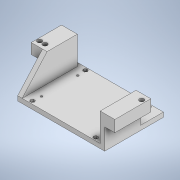
# Autodesk Inventor part: tttray
Saved by Autodesk Inventor 2020 (Build 240168000, 168)
## iProperties
Created: 2022-10-28
Part Number: tttray
Material: 일반
Document SubType Name: Modeling
Designer: SeungJin
Density: 1 g/cm^3
Appearance: 기본값
Author: SeungJin
Autodesk Inventor part; units mm, degrees
ref_plane "YZ Plane" through (0, 0, 0) normal (1, 0, 0) x (0, 1, 0)
ref_plane "XZ Plane" through (0, 0, 0) normal (0, 1, 0) x (-1, 0, 0)
ref_plane "XY Plane" through (0, 0, 0) normal (0, 0, 1) x (1, 0, 0)
sketch "스케치1" plane through (0, 0, 0) normal (0, 1, 0) x (-1, 0, 0)
  line L0 (96.25, 0) -> (-96.25, 0)
  line L1 (-96.25, 0) -> (-96.25, 67)
  line L2 (-96.25, 67) -> (96.25, 67)
  line L3 (96.25, 67) -> (96.25, 0)
  line L4 (96.25, 0) -> (-96.25, 0)
  line L5 (-96.25, 0) -> (-96.25, -63)
  line L6 (-96.25, -63) -> (96.25, -63)
  line L7 (96.25, -63) -> (96.25, 0)
  point P0 (0, 0)
  point P1 (0, 0)
  dimension "d0" = 192.5
  dimension "d1" = 67
  dimension "d2" = 192.5
  dimension "d3" = 63
  constraints: 16 end point, 4 parallel, 2 coincident, 2 horizontal, 2 perpendicular, 1 midpoint
  measures "d0" distance of L1.end L2.end
  measures "d1" distance of L2.end L0.start
  measures "d2" distance of L6.end L5.end
  measures "d3" distance of L6.end L0.start
extrude "돌출1" add sketch "스케치1" along normal blind 10
sketch "스케치2" plane through (0, 10, 0) normal (0, 1, 0) x (1, 0, 0)
  line L0 (-96.25, 0) -> (96.25, 0) projected
  line L1 (-96.25, -67) -> (96.25, -67) projected
  line L2 (86.25, -67) -> (86.25, 12.5)
  line L3 (96.25, -67) -> (96.25, 63) projected
  line L4 (96.25, 12.5) -> (86.25, 12.5)
  line L5 (-86.25, -67) -> (-86.25, 55)
  line L6 (-96.25, 63) -> (-96.25, -67) projected
  line L7 (-96.25, 55) -> (-86.25, 55)
  point P0 (0, 0)
  dimension "d6" = 10
  dimension "d7" = 12.5
  dimension "d8" = 10
  dimension "d9" = 55
  constraints: 8 end point, 4 point on line, 2 perpendicular, 2 vertical
  measures "d6" distance between parallel lines of L2 L3
  measures "d7" distance between parallel lines of L4 L0
  measures "d8" distance between parallel lines of L6 L5
  measures "d9" distance between parallel lines of L7 L0
extrude "돌출2" add sketch "스케치2" along normal blind 62 contours L6 L7 L5 L0 | L0 L5 L1 L6 | L2 L4 L3 L0 | L0 L3 L1 L2
sketch "스케치3" plane through (0, 72, 0) normal (0, 1, 0) x (1, 0, 0)
  line L0 (96.25, -67) -> (96.25, 12.5) projected
  line L1 (96.25, 12.5) -> (86.25, 12.5) projected
  line L2 (86.25, 12.5) -> (86.25, -67) projected
  line L3 (86.25, -67) -> (96.25, -67) projected
  line L4 (96.25, -67) -> (118.75, -67)
  line L5 (118.75, -67) -> (118.75, 12.5)
  line L6 (118.75, 12.5) -> (96.25, 12.5)
  line L7 (96.25, 12.5) -> (96.25, -67)
  point P0 (0, 0)
  dimension "d12" = 22.5
  constraints: 8 end point, 2 parallel, 1 horizontal, 1 perpendicular
  measures "d12" distance of L6.end L5.end
extrude "돌출3" add sketch "스케치3" against normal blind 25.3 contours L0 L6 L5 L4
sketch "스케치5" plane through (0, 72, 0) normal (0, 1, 0) x (1, 0, 0)
  line L0 (-96.25, 55) -> (-96.25, -67) projected
  line L1 (-96.25, -67) -> (-86.25, -67) projected
  line L2 (-86.25, -67) -> (-86.25, 55) projected
  line L3 (-86.25, 55) -> (-96.25, 55) projected
  line L4 (-96.25, 63) -> (-96.25, 55) projected
  line L5 (-96.25, 55) -> (-121.25, 55)
  line L6 (-121.25, 55) -> (-121.25, -12)
  line L7 (-121.25, -12) -> (-96.25, -12)
  line L8 (-96.25, -12) -> (-96.25, 55)
  line L9 (-96.25, 0) -> (96.25, 0) projected
  point P0 (0, 0)
  dimension "d15" = 25
  dimension "d16" = 12
  constraints: 8 end point, 2 parallel, 1 horizontal, 1 perpendicular
  measures "d15" distance between parallel lines of L6 L0
  measures "d16" distance between parallel lines of L9 L7
extrude "돌출4" add sketch "스케치5" against normal blind 23 contours L0 L7 L6 L5
sketch "스케치6" plane through (0, 72, 0) normal (0, 1, 0) x (1, 0, 0)
  line L0 (-96.25, 0) -> (96.25, 0) projected
  line L1 (86.25, 12.5) -> (86.25, -67) projected
  point P0 (0, 0)
  point P1 (111.25, 0)
  point P2 (-114.75, 0)
  point P3 (-102.75, 0)
  dimension "d19" = 25
  dimension "d20" = 214
  dimension "d21" = 12
  measures "d19" distance from line of point (111.25, 0) L1
  measures "d20" distance of point (-102.75, 0) point (111.25, 0)
  measures "d21" distance of point (-114.75, 0) point (-102.75, 0)
hole "구멍1" at (-114.75, 72, 0) at (-102.75, 72, 0) at (111.25, 72, 0) direction (0, -1, 0) diameter 5.5 end through all counterbore diameter 10 counterbore depth 15 clearance for "Socket Head Cap Screw ISO 4762" size "M5" standard "ISO"
sketch "스케치7" plane through (-96.25, 0, -63) normal (-1, 0, 0) x (0, 0, 1)
  line L0 (75, 72) -> (75, 49) projected
  line L1 (75, 49) -> (8, 49) projected
  line L2 (8, 10) -> (8, 49) projected
  line L3 (0, 10) -> (8, 10) projected
  line L4 (0, 0) -> (0, 10) projected
  line L5 (0, 0) -> (130, 0) projected
  line L6 (130, 0) -> (130, 72) projected
  line L7 (75, 72) -> (130, 72) projected
  line L8 (8, 10) -> (130, 10) projected
  line L9 (75, 72) -> (130, 10)
  point P0 (63, 0)
  constraints: 2 end point
extrude "돌출5" cut sketch "스케치7" against normal blind 23 contours L7 L6 L9
sketch "스케치8" plane through (0, 10, 0) normal (0, 1, 0) x (1, 0, 0)
  line L0 (96.25, -67) -> (96.25, 63) projected
  line L1 (-96.25, -67) -> (96.25, -67) projected
  line L2 (-96.25, 63) -> (-96.25, -67) projected
  line L3 (96.25, 63) -> (-96.25, 63) projected
  line L4 (-70, -60.5) -> (70, -60.5)
  line L5 (70, -60.5) -> (70, 56.5)
  line L6 (70, 56.5) -> (-70, 56.5)
  line L7 (-70, 56.5) -> (-70, -60.5)
  line L8 (-70, -60.5) -> (70, 56.5) construction
  line L9 (70, -60.5) -> (-70, 56.5) construction
  circle A0 centre (-70, -60.5) radius 4.15
  circle A1 centre (-70, 56.5) radius 4.15
  circle A2 centre (70, -60.5) radius 4.15
  circle A3 centre (70, 56.5) radius 4.15
  line L10 (-72.396, -64.65) -> (-74.792, -60.5)
  line L11 (-74.792, -60.5) -> (-72.396, -56.35)
  line L12 (-72.396, -56.35) -> (-67.604, -56.35)
  line L13 (-67.604, -56.35) -> (-65.208, -60.5)
  line L14 (-65.208, -60.5) -> (-67.604, -64.65)
  line L15 (-67.604, -64.65) -> (-72.396, -64.65)
  line L16 (-67.604, 60.65) -> (-65.208, 56.5)
  line L17 (-65.208, 56.5) -> (-67.604, 52.35)
  line L18 (-67.604, 52.35) -> (-72.396, 52.35)
  line L19 (-72.396, 52.35) -> (-74.792, 56.5)
  line L20 (-74.792, 56.5) -> (-72.396, 60.65)
  line L21 (-72.396, 60.65) -> (-67.604, 60.65)
  line L22 (67.604, -64.65) -> (65.208, -60.5)
  line L23 (65.208, -60.5) -> (67.604, -56.35)
  line L24 (67.604, -56.35) -> (72.396, -56.35)
  line L25 (72.396, -56.35) -> (74.792, -60.5)
  line L26 (74.792, -60.5) -> (72.396, -64.65)
  line L27 (72.396, -64.65) -> (67.604, -64.65)
  line L28 (72.396, 60.65) -> (74.792, 56.5)
  line L29 (74.792, 56.5) -> (72.396, 52.35)
  line L30 (72.396, 52.35) -> (67.604, 52.35)
  line L31 (67.604, 52.35) -> (65.208, 56.5)
  line L32 (65.208, 56.5) -> (67.604, 60.65)
  line L33 (67.604, 60.65) -> (72.396, 60.65)
  point P0 (0, 0)
  point P1 (0, -2)
  point P2 (0, -2)
  point P3 (-96.25, -2)
  point P4 (-70, -64.65)
  point P5 (-70, 60.65)
  point P6 (70, -64.65)
  point P7 (70, 60.65)
  dimension "d33" = 8.3
  dimension "d34" = 8.3
  dimension "d35" = 8.3
  dimension "d36" = 8.3
  dimension "d31" = 140
  dimension "d32" = 117
  constraints: 60 end point, 8 coincident, 8 midpoint, 4 vertical alignment, 2 parallel, 2 point on line, 1 horizontal, 1 horizontal alignment, 1 perpendicular, 60 other
  measures "d31" distance of L6.end L5.end
  measures "d32" distance of L5.end L4.end
extrude "돌출6" cut sketch "스케치8" against normal blind 5 contours L7 A0 L4 | L4 A0 L7 | A0 L13 L4 | L4 L14 A0 | L12 L13 A0 | A0 L11 L12 | L14 L15 A0 | A1 L6 L7 | L18 L19 A1 | L7 L6 A1 | A1 L17 L18 | A0 L10 L11 | L23 A2 L4 | L4 A2 L22 | L15 L10 A0 | L19 L20 A1 | A1 L6 L17 | A2 L5 L4 | L4 L5 A2 | A2 L27 L22 | L23 L24 A2 | A1 L16 L6 | L20 L21 A1 | A2 L26 L27 | L24 L25 A2 | A1 L21 L16 | L32 A3 L6 | L6 A3 L31 | A2 L25 L26 | A3 L6 L5 | L30 L31 A3 | L5 L6 A3 | A3 L29 L30 | L32 L33 A3 | A3 L28 L29 | L33 L28 A3
sketch "스케치9" plane through (0, 5, 0) normal (0, 1, 0) x (1, 0, 0)
  line L0 (-65.208, -60.5) -> (-67.604, -64.65) projected
  line L1 (-67.604, -56.35) -> (-65.208, -60.5) projected
  line L2 (-72.396, -56.35) -> (-67.604, -56.35) projected
  line L3 (-74.792, -60.5) -> (-72.396, -56.35) projected
  line L4 (-72.396, -64.65) -> (-74.792, -60.5) projected
  line L5 (-67.604, -64.65) -> (-72.396, -64.65) projected
  line L6 (-72.396, 60.65) -> (-67.604, 60.65) projected
  line L7 (-74.792, 56.5) -> (-72.396, 60.65) projected
  line L8 (-72.396, 52.35) -> (-74.792, 56.5) projected
  line L9 (-67.604, 52.35) -> (-72.396, 52.35) projected
  line L10 (-65.208, 56.5) -> (-67.604, 52.35) projected
  line L11 (-67.604, 60.65) -> (-65.208, 56.5) projected
  line L12 (72.396, -56.35) -> (74.792, -60.5) projected
  line L13 (67.604, -56.35) -> (72.396, -56.35) projected
  line L14 (65.208, -60.5) -> (67.604, -56.35) projected
  line L15 (67.604, -64.65) -> (65.208, -60.5) projected
  line L16 (72.396, -64.65) -> (67.604, -64.65) projected
  line L17 (74.792, -60.5) -> (72.396, -64.65) projected
  line L18 (67.604, 52.35) -> (65.208, 56.5) projected
  line L19 (72.396, 52.35) -> (67.604, 52.35) projected
  line L20 (74.792, 56.5) -> (72.396, 52.35) projected
  line L21 (72.396, 60.65) -> (74.792, 56.5) projected
  line L22 (67.604, 60.65) -> (72.396, 60.65) projected
  line L23 (65.208, 56.5) -> (67.604, 60.65) projected
  point P0 (0, 0)
  point P1 (-70, -60.5)
  point P2 (-70, 56.5)
  point P3 (70, -60.5)
  point P4 (70, 56.5)
hole "구멍2" at (-70, 5, 60.5) at (-70, 5, -56.5) at (70, 5, 60.5) at (70, 5, -56.5) direction (0, -1, 0) diameter 5.5 end through all clearance for "Socket Head Cap Screw ISO 4762" size "M5" standard "ISO"
sketch "스케치10" plane through (0, 0, 0) normal (0, -1, 0) x (1, 0, 0)
  circle A0 centre (70, 60.5) radius 2.75 projected
  circle A1 centre (-70, 60.5) radius 2.75 projected
  circle A2 centre (-70, -56.5) radius 2.75 projected
  circle A3 centre (70, -56.5) radius 2.75 projected
  line L0 (96.25, 67) -> (96.25, -63) projected
  line L1 (-96.25, 67) -> (96.25, 67) projected
  line L2 (-96.25, -63) -> (-96.25, 67) projected
  line L3 (96.25, -63) -> (-96.25, -63) projected
  line L4 (68.5, -38) -> (-68.5, -38)
  line L5 (-68.5, -38) -> (-68.5, 42)
  line L6 (-68.5, 42) -> (68.5, 42)
  line L7 (68.5, 42) -> (68.5, -38)
  line L8 (68.5, -38) -> (-68.5, 42) construction
  line L9 (-68.5, -38) -> (68.5, 42) construction
  circle A4 centre (-68.5, -38) radius 3.6
  circle A5 centre (-68.5, 42) radius 3.6
  circle A6 centre (68.5, -38) radius 3.6
  circle A7 centre (68.5, 42) radius 3.6
  line L10 (-70.5785, -41.6) -> (-72.6569, -38)
  line L11 (-72.6569, -38) -> (-70.5785, -34.4)
  line L12 (-70.5785, -34.4) -> (-66.4215, -34.4)
  line L13 (-66.4215, -34.4) -> (-64.3431, -38)
  line L14 (-64.3431, -38) -> (-66.4215, -41.6)
  line L15 (-66.4215, -41.6) -> (-70.5785, -41.6)
  line L16 (-70.5785, 38.4) -> (-72.6569, 42)
  line L17 (-72.6569, 42) -> (-70.5785, 45.6)
  line L18 (-70.5785, 45.6) -> (-66.4215, 45.6)
  line L19 (-66.4215, 45.6) -> (-64.3431, 42)
  line L20 (-64.3431, 42) -> (-66.4215, 38.4)
  line L21 (-66.4215, 38.4) -> (-70.5785, 38.4)
  line L22 (66.4215, 38.4) -> (64.3431, 42)
  line L23 (64.3431, 42) -> (66.4215, 45.6)
  line L24 (66.4215, 45.6) -> (70.5785, 45.6)
  line L25 (70.5785, 45.6) -> (72.6569, 42)
  line L26 (72.6569, 42) -> (70.5785, 38.4)
  line L27 (70.5785, 38.4) -> (66.4215, 38.4)
  line L28 (70.5785, -34.4) -> (72.6569, -38)
  line L29 (72.6569, -38) -> (70.5785, -41.6)
  line L30 (70.5785, -41.6) -> (66.4215, -41.6)
  line L31 (66.4215, -41.6) -> (64.3431, -38)
  line L32 (64.3431, -38) -> (66.4215, -34.4)
  line L33 (66.4215, -34.4) -> (70.5785, -34.4)
  point P0 (0, 0)
  point P1 (0, 2)
  point P2 (-68.5, 2)
  point P3 (-96.25, 2)
  point P4 (0, 2)
  point P5 (-68.5, -41.6)
  point P6 (-68.5, 38.4)
  point P7 (68.5, 38.4)
  point P8 (68.5, -34.4)
  dimension "d48" = 7.2
  dimension "d49" = 7.2
  dimension "d50" = 7.2
  dimension "d51" = 7.2
  dimension "d46" = 137
  dimension "d47" = 80
  constraints: 60 end point, 9 midpoint, 7 coincident, 5 vertical alignment, 3 point on line, 2 parallel, 1 horizontal, 1 horizontal alignment, 1 perpendicular, 60 other
  measures "d46" distance of L5.end L6.end
  measures "d47" distance of L4.end L5.end
extrude "돌출7" cut sketch "스케치10" against normal blind 5 contours L32 A6 L4 | L4 A6 L31 | L14 A4 L4 | L4 A4 L13 | A6 L7 L4 | L4 L7 A6 | A6 L30 L31 | L32 L33 A6 | A4 L5 L4 | L4 L5 A4 | A4 L12 L13 | L14 L15 A4 | A6 L29 L30 | L33 L28 A6 | A4 L11 L12 | L15 L10 A4 | A6 L28 L29 | A7 L6 L7 | L27 L22 A7 | L7 L6 A7 | A7 L26 L27 | A5 L6 L5 | L21 L16 A5 | L5 L6 A5 | A5 L20 L21 | A4 L10 L11 | L22 L6 A7 | A7 L25 L26 | L16 L17 A5 | A5 L6 L20 | L6 L23 A7 | A5 L19 L6 | L17 L18 A5 | L23 L24 A7 | A7 L24 L25 | A5 L18 L19
sketch "스케치11" plane through (0, 5, 0) normal (0, -1, 0) x (1, 0, 0)
  line L0 (-64.3431, -38) -> (-66.4215, -41.6) projected
  line L1 (-66.4215, -34.4) -> (-64.3431, -38) projected
  line L2 (-70.5785, -34.4) -> (-66.4215, -34.4) projected
  line L3 (-72.6569, -38) -> (-70.5785, -34.4) projected
  line L4 (-70.5785, -41.6) -> (-72.6569, -38) projected
  line L5 (-66.4215, -41.6) -> (-70.5785, -41.6) projected
  line L6 (-66.4215, 45.6) -> (-64.3431, 42) projected
  line L7 (-70.5785, 45.6) -> (-66.4215, 45.6) projected
  line L8 (-72.6569, 42) -> (-70.5785, 45.6) projected
  line L9 (-70.5785, 38.4) -> (-72.6569, 42) projected
  line L10 (-66.4215, 38.4) -> (-70.5785, 38.4) projected
  line L11 (-64.3431, 42) -> (-66.4215, 38.4) projected
  line L12 (72.6569, 42) -> (70.5785, 38.4) projected
  line L13 (70.5785, 45.6) -> (72.6569, 42) projected
  line L14 (66.4215, 45.6) -> (70.5785, 45.6) projected
  line L15 (64.3431, 42) -> (66.4215, 45.6) projected
  line L16 (66.4215, 38.4) -> (64.3431, 42) projected
  line L17 (70.5785, 38.4) -> (66.4215, 38.4) projected
  line L18 (70.5785, -34.4) -> (72.6569, -38) projected
  line L19 (66.4215, -34.4) -> (70.5785, -34.4) projected
  line L20 (64.3431, -38) -> (66.4215, -34.4) projected
  line L21 (66.4215, -41.6) -> (64.3431, -38) projected
  line L22 (70.5785, -41.6) -> (66.4215, -41.6) projected
  line L23 (72.6569, -38) -> (70.5785, -41.6) projected
  point P0 (0, 0)
  point P1 (-68.5, -38)
  point P2 (-68.5, 42)
  point P3 (68.5, 42)
  point P4 (68.5, -38)
hole "구멍3" at (-68.5, 5, -38) at (-68.5, 5, 42) at (68.5, 5, 42) at (68.5, 5, -38) direction (0, 1, 0) diameter 4.5 end through all clearance for "Socket Head Cap Screw ISO 4762" size "M4" standard "ISO"
